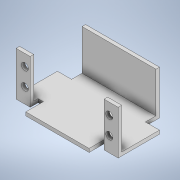
# Autodesk Inventor part: Деталь4
Saved by Autodesk Inventor 2020.1 (Build 241239000, 239)
## iProperties
Created: 2021-08-12
Part Number: Деталь4
Material: Типовые
Document SubType Name: Modeling
Designer: User
Density: 1 g/cm^3
Appearance: По умолчанию
Author: User
Autodesk Inventor part; units mm, degrees
ref_plane "YZ Plane" through (0, 0, 0) normal (1, 0, 0) x (0, 1, 0)
ref_plane "XZ Plane" through (0, 0, 0) normal (0, 1, 0) x (-1, 0, 0)
ref_plane "XY Plane" through (0, 0, 0) normal (0, 0, 1) x (1, 0, 0)
sketch "Эскиз2" plane through (0, 0, 0) normal (0, 1, 0) x (-1, 0, 0)
  line L0 (0, 0) -> (-58, 0)
  line L1 (-58, 0) -> (-58, 37)
  line L2 (-58, 37) -> (0, 37)
  line L3 (0, 37) -> (0, 0)
  line L4 (-58, 8) -> (-50, 8)
  line L5 (-50, 8) -> (-50, 0)
  line L6 (-50, 0) -> (-58, 0)
  line L7 (-58, 0) -> (-58, 8)
  line L8 (-58, 37) -> (-47, 37)
  line L9 (-47, 37) -> (-47, 27)
  line L10 (-47, 27) -> (-58, 27)
  line L11 (-58, 27) -> (-58, 37)
  line L12 (-50, 27) -> (-58, 27)
  line L13 (-58, 27) -> (-58, 31.5)
  line L14 (-58, 31.5) -> (-50, 31.5)
  line L15 (-50, 31.5) -> (-50, 27)
  line L16 (0, 37) -> (-11, 37)
  line L17 (-11, 37) -> (-11, 27)
  line L18 (-11, 27) -> (0, 27)
  line L19 (0, 27) -> (0, 37)
  line L20 (-11, 27) -> (-7.6324, 27)
  line L21 (-11, 31.5) -> (-11, 27)
  line L22 (0, 27) -> (-8, 27)
  line L23 (-8, 27) -> (-8, 31.5)
  line L24 (-8, 31.5) -> (0, 31.5)
  line L25 (0, 31.5) -> (0, 27)
  line L26 (-8, 8) -> (0, 8)
  line L27 (0, 8) -> (0, 0)
  line L28 (0, 0) -> (-8, 0)
  line L29 (-8, 0) -> (-8, 8)
  point P0 (0, 31.5)
  dimension "d0" = 58
  dimension "d1" = 37
  dimension "d2" = 8
  dimension "d3" = 8
  dimension "d4" = 10
  dimension "d5" = 11
  dimension "d6" = 4.5
  dimension "d7" = 10
  dimension "d8" = 11
  dimension "d9" = 8
  constraints: 60 end point, 14 parallel, 8 horizontal, 7 perpendicular, 4 point on line
  measures "d0" distance of L0.start L0.end
  measures "d1" distance of L2.end L0.start
  measures "d2" distance of L4.start L4.end
  measures "d3" distance of L4.end L5.end
  measures "d4" distance of L8.end L9.end
  measures "d5" distance of L9.end L10.end
  measures "d6" distance of L14.end L12.start
  measures "d7" distance of L16.end L17.end
  measures "d8" distance of L17.end L18.end
  measures "d9" distance of L23.end L24.end
extrude "Выдавливание1" add sketch "Эскиз2" along normal blind 2 contours L0 L5 L4 L1 L10 L9 L2 L17 L18 L3 L26 L29 | L18 L23 L24 L3 | L1 L14 L15 L10
sketch "Эскиз3" plane through (0, 2, 0) normal (0, 1, 0) x (1, 0, 0)
  line L0 (0, -31.5) -> (8, -31.5) projected
  line L1 (0, -8) -> (0, -31.5) projected
  line L2 (8, -31.5) -> (0, -31.5)
  line L3 (0, -31.5) -> (0, -29.5)
  line L4 (0, -29.5) -> (8, -29.5)
  line L5 (8, -29.5) -> (8, -31.5)
  line L6 (50, -31.5) -> (58, -31.5) projected
  line L7 (58, -31.5) -> (58, -8) projected
  line L8 (50, -31.5) -> (58, -31.5)
  line L9 (58, -31.5) -> (58, -29.5)
  line L10 (58, -29.5) -> (50, -29.5)
  line L11 (50, -29.5) -> (50, -31.5)
  line L12 (50, 0) -> (8, 0) projected
  line L13 (8, 0) -> (8, -8) projected
  line L14 (50, 0) -> (8, 0)
  line L15 (8, 0) -> (8, -2)
  line L16 (8, -2) -> (50, -2)
  line L17 (50, -2) -> (50, 0)
  point P0 (0, 0)
  dimension "d12" = 2
  dimension "d13" = 2
  constraints: 24 end point, 6 parallel, 3 horizontal, 3 perpendicular, 3 point on line
  measures "d12" distance of L0.end L4.end
  measures "d13" distance from line of L12 L15.end
extrude "Выдавливание2" add sketch "Эскиз3" along normal blind 23
sketch "Эскиз4" plane through (50, 0, 31.5) normal (0, 0, 1) x (1, 0, 0)
  line L0 (-42, 2) -> (-50, 2) projected
  line L1 (-42, 0) -> (-42, 25) projected
  line L2 (-42, 2) -> (-42, 25)
  line L3 (0, 0) -> (0, 25) projected
  circle A0 centre (-45, 18.5) radius 2
  circle A1 centre (-45, 8.5) radius 2
  circle A2 centre (3, 18.5) radius 2
  circle A3 centre (3, 8.5) radius 2
  point P0 (-50, 0)
  point P1 (-42, 13.5)
  point P2 (0, 13.5)
  dimension "d16" = 4
  dimension "d17" = 5
  dimension "d18" = 3
  dimension "d19" = 4
  dimension "d20" = 5
  dimension "d21" = 4
  dimension "d22" = 5
  dimension "d23" = 3
  dimension "d24" = 4
  constraints: 4 centre point, 2 end point, 1 collinear, 1 midpoint, 1 point on line
  measures "d16" diameter of A0
  measures "d17" vertical distance of A0.centre point (-42, 13.5)
  measures "d18" horizontal distance of A0.centre point (-42, 13.5)
  measures "d19" diameter of A1
  measures "d20" vertical distance of point (-42, 13.5) A1.centre
  measures "d21" diameter of A2
  measures "d22" vertical distance of A2.centre point (0, 13.5)
  measures "d23" distance from line of L3 A2.centre
  measures "d24" diameter of A3
extrude "Выдавливание3" cut sketch "Эскиз4" against normal blind 10
